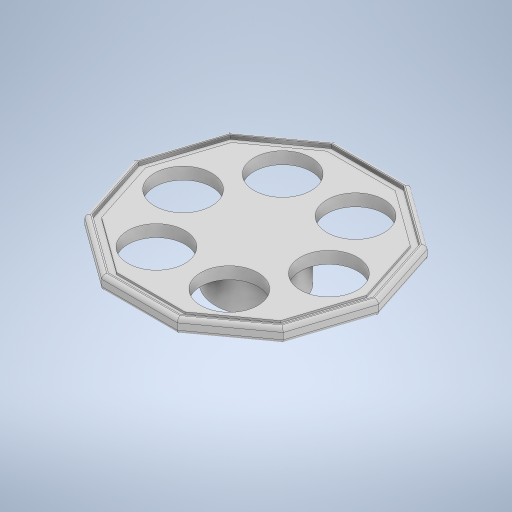
# Autodesk Inventor part: OV-PAM_n_10_bottom
Saved by Autodesk Inventor 2024 (Build 280153000, 153)
## iProperties
Created: 2023-08-31
Part Number: OV-PAM_n_10_bottom
Material: 일반
Document SubType Name: Modeling
Designer: jsw
Density: 1 g/cm^3
Appearance: 기본값
Author: jsw
Autodesk Inventor part; units mm, degrees
ref_plane "YZ Plane" through (0, 0, 0) normal (1, 0, 0) x (0, 1, 0)
ref_plane "XZ Plane" through (0, 0, 0) normal (0, 1, 0) x (-1, 0, 0)
ref_plane "XY Plane" through (0, 0, 0) normal (0, 0, 1) x (1, 0, 0)
sketch "스케치1" plane through (0, 0, 0) normal (0, 1, 0) x (-1, 0, 0)
  line L0 (-10.9012, 33.5504) -> (10.9012, 33.5504)
  line L1 (10.9012, 33.5504) -> (28.5397, 20.7353)
  line L2 (28.5397, 20.7353) -> (35.277, 0)
  line L3 (35.277, 0) -> (28.5397, -20.7353)
  line L4 (28.5397, -20.7353) -> (10.9012, -33.5504)
  line L5 (10.9012, -33.5504) -> (-10.9012, -33.5504)
  line L6 (-10.9012, -33.5504) -> (-28.5397, -20.7353)
  line L7 (-28.5397, -20.7353) -> (-35.277, 0)
  line L8 (-35.277, 0) -> (-28.5397, 20.7353)
  line L9 (-28.5397, 20.7353) -> (-10.9012, 33.5504)
  line L10 (11.9409, -36.7504) -> (-11.9409, -36.7504)
  line L11 (-11.9409, -36.7504) -> (-31.2618, -22.713)
  line L12 (-31.2618, -22.713) -> (-38.6417, 0)
  line L13 (-38.6417, 0) -> (-31.2618, 22.713)
  line L14 (-31.2618, 22.713) -> (-11.9409, 36.7504)
  line L15 (-11.9409, 36.7504) -> (11.9409, 36.7504)
  line L16 (11.9409, 36.7504) -> (31.2618, 22.713)
  line L17 (31.2618, 22.713) -> (38.6417, 0)
  line L18 (38.6417, 0) -> (31.2618, -22.713)
  line L19 (31.2618, -22.713) -> (11.9409, -36.7504)
  point P0 (0, 0)
  point P1 (0, 0)
  point P2 (0, 0)
  dimension "d0" = 70.554
  dimension "d1" = 3.2
  constraints: 40 end point, 2 coincident, 2 horizontal, 42 other
  measures "d0" distance of L7.end L2.end
  measures "d1" distance between parallel lines of L3 L18
extrude "돌출1" add sketch "스케치1" along normal blind 4.4 contours L0 L1 L2 L3 L4 L5 L6 L7 L8 L9 | L10 L11 L12 L13 L14 L15 L16 L17 L18 L19
sketch "스케치2" plane through (0, 4.4, 0) normal (0, 1, 0) x (1, 0, 0)
  line L0 (-11.4211, 35.1504) -> (11.4211, 35.1504)
  line L1 (11.4211, 35.1504) -> (29.9007, 21.7242)
  line L2 (29.9007, 21.7242) -> (36.9593, 0)
  line L3 (36.9593, 0) -> (29.9007, -21.7242)
  line L4 (29.9007, -21.7242) -> (11.4211, -35.1504)
  line L5 (11.4211, -35.1504) -> (-11.4211, -35.1504)
  line L6 (-11.4211, -35.1504) -> (-29.9007, -21.7242)
  line L7 (-29.9007, -21.7242) -> (-36.9593, 0)
  line L8 (-36.9593, 0) -> (-29.9007, 21.7242)
  line L9 (-29.9007, 21.7242) -> (-11.4211, 35.1504)
  line L10 (-31.2618, 22.713) -> (-38.6417, 0) projected
  point P0 (0, 0)
  point P1 (0, 0)
  dimension "d4" = 1.6
  constraints: 20 end point, 1 coincident, 1 horizontal, 21 other
  measures "d4" distance between parallel lines of L8 L10
extrude "돌출2" cut sketch "스케치2" against normal blind 1.2
sketch "스케치3" plane through (0, 3.2, 0) normal (0, 1, 0) x (1, 0, 0)
  line L0 (-10.7712, 33.1504) -> (10.7712, 33.1504)
  line L1 (10.7712, 33.1504) -> (28.1994, 20.4881)
  line L2 (28.1994, 20.4881) -> (34.8564, 0)
  line L3 (34.8564, 0) -> (28.1994, -20.4881)
  line L4 (28.1994, -20.4881) -> (10.7712, -33.1504)
  line L5 (10.7712, -33.1504) -> (-10.7712, -33.1504)
  line L6 (-10.7712, -33.1504) -> (-28.1994, -20.4881)
  line L7 (-28.1994, -20.4881) -> (-34.8564, 0)
  line L8 (-34.8564, 0) -> (-28.1994, 20.4881)
  line L9 (-28.1994, 20.4881) -> (-10.7712, 33.1504)
  line L10 (-29.9007, 21.7242) -> (-11.4211, 35.1504) projected
  point P0 (0, 0)
  point P1 (0, 0)
  dimension "d7" = 2
  constraints: 20 end point, 1 coincident, 1 horizontal, 21 other
  measures "d7" distance between parallel lines of L10 L9
extrude "돌출3" add sketch "스케치3" along normal blind 0.6
fillet "모깎기1" radius 1.2 20 edges at (0, 4.4, 36.7504) (0, 0, 36.7504) (-21.6014, 4.4, 29.7317) (-21.6014, 0, 29.7317) (-34.9517, 4.4, 11.3565) (-34.9517, 4.4, -11.3565) (-21.6014, 4.4, -29.7317) (0, 4.4, -36.7504) (21.6014, 4.4, -29.7317) (34.9517, 4.4, -11.3565) (34.9517, 4.4, 11.3565) (21.6014, 4.4, 29.7317) (21.6014, 0, -29.7317) (0, 0, -36.7504) (-21.6014, 0, -29.7317) (-34.9517, 0, -11.3565) (-34.9517, 0, 11.3565) (34.9517, 0, -11.3565) (34.9517, 0, 11.3565) (21.6014, 0, 29.7317)
sketch "스케치12" plane through (0, 0, 0) normal (0, -1, 0) x (1, 0, 0)
  circle A0 centre (0, 0) radius 12.7
  dimension "d53" = 25.4
  constraints: 1 centre point, 1 coincident
  measures "d53" diameter of A0
extrude "돌출12" add sketch "스케치12" along normal blind 10.16
sketch "스케치13" plane through (0, -10.16, 0) normal (0, -1, 0) x (1, 0, 0)
  circle A0 centre (0, 0) radius 4.5
  line L0 (-2.5981, 4.5) -> (2.5981, 4.5)
  line L1 (2.5981, 4.5) -> (5.1962, 0)
  line L2 (5.1962, 0) -> (2.5981, -4.5)
  line L3 (2.5981, -4.5) -> (-2.5981, -4.5)
  line L4 (-2.5981, -4.5) -> (-5.1962, 0)
  line L5 (-5.1962, 0) -> (-2.5981, 4.5)
  point P0 (-3.8971, 2.25)
  point P1 (-3.8971, -2.25)
  point P2 (0, 4.5)
  point P3 (0, -4.5)
  point P4 (3.8971, -2.25)
  point P5 (3.8971, 2.25)
  dimension "d56" = 9
  constraints: 12 end point, 2 coincident, 1 centre point, 1 horizontal, 1 tangent, 13 other
  measures "d56" diameter of A0
extrude "돌출13" cut sketch "스케치13" against normal blind 12
sketch "스케치14" plane through (0, 0, 0) normal (0, -1, 0) x (1, 0, 0)
  circle A0 centre (-23, 0) radius 9
  circle A1 centre (-11.5, -19.9186) radius 9
  circle A2 centre (11.5, -19.9186) radius 9
  circle A3 centre (23, 0) radius 9
  circle A4 centre (11.5, 19.9186) radius 9
  circle A5 centre (-11.5, 19.9186) radius 9
  point P0 (0, 0)
  dimension "d61" = 18
  dimension "d62" = 23
  dimension "d65" = 360
  constraints: 6 centre point, 1 horizontal alignment, 13 other
  measures "d61" diameter of A0
  measures "d62" distance of A0.centre point (0, 0)
extrude "돌출14" cut sketch "스케치14" against normal up to surface (3.8 mm away)
sketch "스케치17" plane through (0, 1.84, 0) normal (0, -1, 0) x (1, 0, 0)
  line L0 (-2.5981, 4.5) -> (2.5981, 4.5) projected
  line L1 (-5.1962, 0) -> (-2.5981, 4.5) projected
  line L2 (-2.5981, -4.5) -> (-5.1962, 0) projected
  line L3 (2.5981, -4.5) -> (-2.5981, -4.5) projected
  line L4 (5.1962, 0) -> (2.5981, -4.5) projected
  line L5 (2.5981, 4.5) -> (5.1962, 0) projected
  line L6 (-2.0207, 3.5) -> (2.0207, 3.5)
  line L7 (2.0207, 3.5) -> (4.0415, 0)
  line L8 (4.0415, 0) -> (2.0207, -3.5)
  line L9 (2.0207, -3.5) -> (-2.0207, -3.5)
  line L10 (-2.0207, -3.5) -> (-4.0415, 0)
  line L11 (-4.0415, 0) -> (-2.0207, 3.5)
  point P0 (0, 0)
  point P1 (0, 0)
  dimension "d87" = 1
  constraints: 12 end point, 1 coincident, 1 horizontal, 13 other
  measures "d87" distance between parallel lines of L6 L0
extrude "돌출15" add sketch "스케치17" along normal blind 8.5
fillet "모깎기2" radius 0.5 6 edges at (0, -10.16, 4.5) (-3.8971, -10.16, 2.25) (-3.8971, -10.16, -2.25) (3.8971, -10.16, 2.25) (3.8971, -10.16, -2.25) (0, -10.16, -4.5)
equation "\"d76\" = 55deg"
